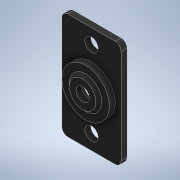
# Autodesk Inventor part: LinearActuatorHolder
Saved by Autodesk Inventor 2021 (Build 250183000, 183)
## iProperties
Created: 2020-07-16
Part Number: LinearActuatorHolder
Material: Generic
Document SubType Name: Modeling
Designer: CASE-SMALL2
Density: 1 g/cm^3
Appearance: Default
Author: CASE-SMALL2
Autodesk Inventor part; units mm, degrees
ref_plane "YZ Plane" through (0, 0, 0) normal (1, 0, 0) x (0, 1, 0)
ref_plane "XZ Plane" through (0, 0, 0) normal (0, 1, 0) x (-1, 0, 0)
ref_plane "XY Plane" through (0, 0, 0) normal (0, 0, 1) x (1, 0, 0)
sketch "Sketch4" plane through (0, 0, 0) normal (0, 0, 1) x (1, 0, 0)
  line L0 (-10, -18) -> (10, -18)
  line L1 (10, -18) -> (10, 18)
  line L2 (10, 18) -> (-10, 18)
  line L3 (-10, 18) -> (-10, -18)
  line L4 (-10, -18) -> (10, 18) construction
  line L5 (10, -18) -> (-10, 18) construction
  point P0 (0, 0)
  dimension "d16" = 20
  dimension "d17" = 36
  constraints: 12 end point, 2 midpoint, 2 parallel, 1 horizontal, 1 perpendicular
  measures "d16" distance of L1.end L2.end
  measures "d17" distance of L0.end L1.end
extrude "Extrusion4" add sketch "Sketch4" along normal blind 2
sketch "Sketch5" plane through (0, 0, 2) normal (0, 0, 1) x (1, 0, 0)
  line L0 (0, 25.2) -> (0, -25.2) projected
  circle A0 centre (0, 13) radius 2.25
  circle A1 centre (0, -13) radius 2.25
  line L1 (10, 18) -> (-10, 18) projected
  line L2 (-10, -18) -> (10, -18) projected
  point P0 (0, 0)
  dimension "d20" = 4.5
  dimension "d21" = 4.5
  dimension "d22" = 5
  dimension "d23" = 5
  constraints: 2 centre point, 2 point on line
  measures "d20" diameter of A0
  measures "d21" diameter of A1
  measures "d22" distance from line of L1 A0.centre
  measures "d23" distance from line of L2 A1.centre
extrude "Extrusion5" cut sketch "Sketch5" against normal through all
sketch "Sketch6" plane through (0, 0, 2) normal (0, 0, 1) x (1, 0, 0)
  circle A0 centre (0, 0) radius 8
  dimension "d26" = 16
  constraints: 1 centre point, 1 coincident
  measures "d26" diameter of A0
extrude "Extrusion6" add sketch "Sketch6" along normal blind 2
fillet "Fillet1" radius 2 4 edges at (10, 18, 1) (-10, 18, 1) (-10, -18, 1) (10, -18, 1)
sketch "Sketch7" plane through (0, 0, 4) normal (0, 0, 1) x (1, 0, 0)
  circle A0 centre (0, 0) radius 3.5
  dimension "d30" = 7
  constraints: 1 centre point, 1 coincident
  measures "d30" diameter of A0
extrude "Extrusion7" add sketch "Sketch7" along normal blind 6
chamfer "Chamfer1" distance 2 angle 45 1 edges at (-3.5, 0, 4)
sketch "Sketch8" plane through (0, 0, 10) normal (0, 0, 1) x (1, 0, 0)
  circle A0 centre (0, 0) radius 2.25
  dimension "d36" = 4.5
  constraints: 1 centre point, 1 coincident
  measures "d36" diameter of A0
extrude "Extrusion8" cut sketch "Sketch8" against normal through all
chamfer "Chamfer2" distance 3 angle 45 1 edges at (-2.25, 0, 0)
sketch "Sketch10" plane through (0, 0, 10) normal (0, 0, 1) x (1, 0, 0)
  circle A0 centre (0, 0) radius 13.6126
  constraints: 1 centre point, 1 coincident
extrude "Extrusion9" cut sketch "Sketch10" against normal blind 5
equation "\"d21\" = d20"
equation "\"d23\" = d22"
body "Solid2"
